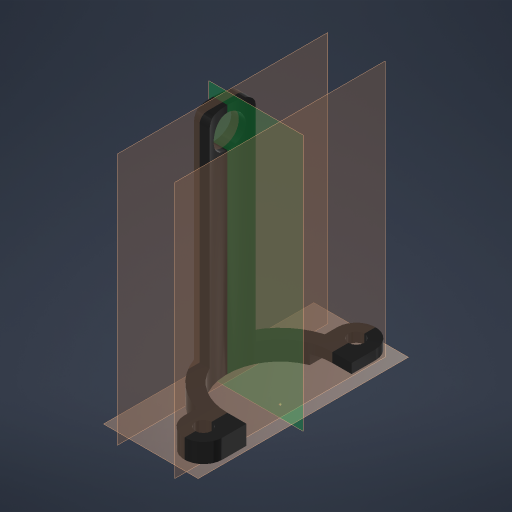
# Autodesk Inventor part: Tube Holder V2
Saved by Autodesk Inventor 2024 (Build 280153000, 153)
## iProperties
Manager: Louis Van Roosmaelen
Company: DCS - DIGITAL COMBAT SIMULATOR
Created: 2023-11-03
Part Number: Tube Holder V2
Material: S235
Catalog Web Link: http://emmausbovenbouw.op-weg.be/
Vendor: Emmaüsinstituut Bovenbouw Aalter
Document SubType Name: Modeling
Designer: Louis
Engineer: Declercq St.
Manufacturer: Standard
Standards Organization: Custom
Density: 7.86 g/cm^3
Appearance: Smooth - Black
IDENT.NR.: AJ2022
TEAM: 30
Title: F18C Home Cockpit
Author: Louis
Keywords: Ø
Autodesk Inventor part; units mm, degrees
sketch "Sketch1" plane through (0, 0, 0) normal (0, 0, 1) x (1, 0, 0)
  line L0 (0, 2.8582) -> (0, -2.8582) construction
  line L1 (-5.7775, 0) -> (5.7775, 0) construction
  arc A0 (0, 17.5) -> (0, -17.5) centre (0, 0) ccw
  arc A1 (0, 13.75) -> (0, -13.75) centre (0, 0) ccw
  line L2 (0, 35) -> (0, -35) construction
  line L3 (5, 25) -> (5, 17.5)
  line L4 (-5, 16.7705) -> (-5, 25)
  line L5 (-5, 25) -> (5, 25)
  line L6 (-5, -16.7705) -> (-5, -25)
  line L7 (-5, -25) -> (5, -25)
  line L8 (0, 17.5) -> (5, 17.5)
  line L9 (5, -25) -> (5, -23.6416)
  line L10 (5, -23.6416) -> (5, -13.75)
  line L11 (5, -13.75) -> (0, -13.75)
  line L12 (0, -17.5) -> (5, -17.5)
  line L13 (0, 13.75) -> (5, 13.75)
  line L14 (5, 13.75) -> (5, 17.5)
  point P0 (0, 20)
  point P1 (0, -20)
  dimension "d0" = 35
  dimension "d1" = 27.5
  dimension "d2" = 20
  dimension "d3" = 20
  dimension "d4" = 10
  dimension "d5" = 5
  dimension "d6" = 5
  constraints: 28 end point, 5 point on circle, 4 perpendicular, 3 coincident, 3 symmetric about line, 3 vertical, 2 centre point, 2 horizontal, 2 midpoint, 2 point on line, 2 tangent, 1 collinear, 7 other
  measures "d0" diameter of A0
  measures "d1" diameter of A1
  measures "d2" distance from line of L1 point (0, -20)
  measures "d3" distance from line of L1 point (0, 20)
  measures "d4" distance of L4.end L3.start
  measures "d5" distance from line of point (0, 20) L5
  measures "d6" distance from line of point (0, 20) L3
extrude "Extrusion1" add sketch "Sketch1" along normal blind 5
sketch "Sketch2" plane through (0, 0, 5) normal (0, 0, 1) x (1, 0, 0)
  line L0 (5, 25) -> (5, 13.75) projected
  line L1 (5, 13.75) -> (0, 13.75) projected
  arc A0 (0, 13.75) -> (0, -13.75) centre (0, 0) ccw projected
  line L2 (0, -13.75) -> (5, -13.75) projected
  line L3 (5, -13.75) -> (5, -25) projected
  line L4 (5, -25) -> (-5, -25) projected
  line L5 (-5, -25) -> (-5, -16.7705) projected
  arc A1 (-5, 16.7705) -> (-5, -16.7705) centre (0, 0) ccw projected
  line L6 (-5, 16.7705) -> (-5, 25) projected
  line L7 (-5, 25) -> (5, 25) projected
  point P0 (0, 20)
  point P1 (0, -20)
  dimension "d9" = 5
  dimension "d10" = 5
  dimension "d11" = 5
  dimension "d12" = 5
  measures "d9" distance from line of L4 point (0, -20)
  measures "d10" distance from line of point (0, -20) L5
  measures "d11" distance from line of L6 point (0, 20)
  measures "d12" distance from line of L7 point (0, 20)
hole "Hole1" at (0, 20, 5) at (0, -20, 5) direction (0, 0, -1) diameter 4.2 end through all
fillet "Fillet1" radius 5 4 edges at (-5, -25, 2.5) (5, -25, 2.5) (5, 25, 2.5) (-5, 25, 2.5)
sketch "Sketch3" plane through (0, 0, 0) normal (0, 0, -1) x (-1, 0, 0)
  circle A0 centre (0, -20) radius 2.1 projected
  circle A1 centre (0, 20) radius 2.1 projected
  arc A2 (5, 20) -> (-5, 20) centre (0, 20) ccw projected
  line L0 (5, 20) -> (5, 16.7705) projected
  arc A3 (5, -16.7705) -> (5, 16.7705) centre (0, 0) ccw projected
  line L1 (5, -16.7705) -> (5, -20) projected
  arc A4 (-5, -20) -> (5, -20) centre (0, -20) ccw projected
  line L2 (-5, -20) -> (-5, -13.75) projected
  line L3 (-5, -13.75) -> (0, -13.75) projected
  arc A5 (0, -13.75) -> (0, 13.75) centre (0, 0) ccw projected
  line L4 (0, 13.75) -> (-5, 13.75) projected
  line L5 (-5, 13.75) -> (-5, 20) projected
  line L6 (5, 16.7705) -> (5, 12.8087)
  constraints: 2 end point, 1 point on circle, 1 vertical
extrude "Extrusion2" cut sketch "Sketch3" against normal blind 2.5 contours L0 L6 A5 L4 L5 A2
sketch "Sketch4" plane through (0, 0, 5) normal (0, 0, 1) x (1, 0, 0)
  arc A0 (-5, -20) -> (5, -20) centre (0, -20) ccw projected
  line L0 (-5, -20) -> (-5, -16.7705) projected
  arc A1 (-5, 16.7705) -> (-5, -16.7705) centre (0, 0) ccw projected
  line L1 (-5, 16.7705) -> (-5, 20) projected
  arc A2 (5, 20) -> (-5, 20) centre (0, 20) ccw projected
  line L2 (5, 20) -> (5, 13.75) projected
  line L3 (5, 13.75) -> (0, 13.75) projected
  arc A3 (0, 13.75) -> (0, -13.75) centre (0, 0) ccw projected
  line L4 (0, -13.75) -> (5, -13.75) projected
  line L5 (5, -13.75) -> (5, -20) projected
  circle A4 centre (0, -20) radius 2.1 projected
  circle A5 centre (0, 20) radius 2.1 projected
  line L6 (-16.4393, -6) -> (-12.3718, -6)
  line L7 (-16.4393, 6) -> (-12.3718, 6)
  line L8 (-22, 0) -> (9.5, 0) construction
  dimension "d23" = 12
  dimension "d24" = 6
  constraints: 4 end point, 4 point on circle, 2 horizontal
  measures "d23" distance between parallel lines of L7 L6
  measures "d24" distance between parallel lines of L8 L7
extrude "Extrusion3" add sketch "Sketch4" along normal blind 56 contours A1 L7 A3 L6
ref_plane "Work Plane1" through (-15, 0, 0) normal (1, 0, 0) x (0, 1, 0)
sketch "Sketch5" plane through (-15, 0, 0) normal (1, 0, 0) x (0, 1, 0)
  line L0 (9.0139, 0) -> (-9.0139, 0) projected
  line L1 (-9.0139, 0) -> (-9.0139, 5) projected
  line L2 (-9.0139, 5) -> (-6, 5) projected
  line L3 (-6, 5) -> (-6, 61) projected
  line L4 (-6, 61) -> (6, 61) projected
  line L5 (6, 61) -> (6, 5) projected
  line L6 (6, 5) -> (9.0139, 5) projected
  line L7 (9.0139, 5) -> (9.0139, 0) projected
  circle A0 centre (0, 55) radius 4.25
  point P0 (0, 0)
  dimension "d30" = 55
  constraints: 1 centre point
  measures "d30" distance from line of L0 A0.centre
extrude "Extrusion4" cut sketch "Sketch5" along normal through all both and the other way through all contours A0
fillet "Fillet2" radius 2 2 edges at (-14.4056, -6, 61) (-14.4056, 6, 61)
equation "\"d24\" = 0.5 * d23"
body "Solid1"
